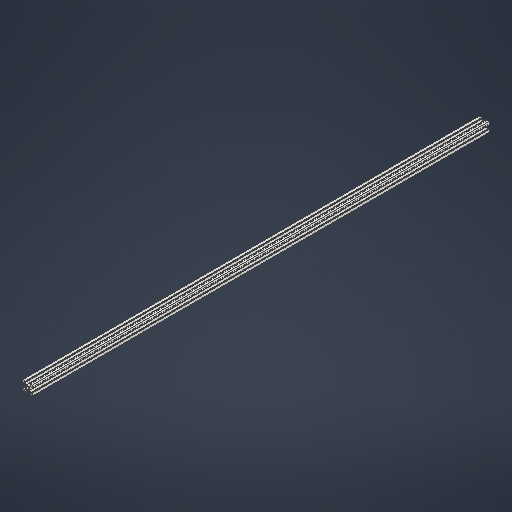
# Autodesk Inventor part: 铝方管2020x
Saved by Autodesk Inventor 2025 (Build 290162000, 162)
## iProperties
Created: 2025-06-18
Part Number: 铝方管2020x
Material: 常规
Document SubType Name: Modeling
Designer: XH
Density: 1 g/cm^3
Appearance: 默认
Author: XH
Autodesk Inventor part; units mm, degrees
ref_plane "YZ Plane" through (0, 0, 0) normal (1, 0, 0) x (0, 1, 0)
ref_plane "XZ Plane" through (0, 0, 0) normal (0, 1, 0) x (-1, 0, 0)
ref_plane "XY Plane" through (0, 0, 0) normal (0, 0, 1) x (1, 0, 0)
sketch "草图1" plane through (0, 0, 0) normal (0, 0, 1) x (1, 0, 0)
  line L0 (10, -10) -> (-10, -10)
  line L1 (-10, -10) -> (-10, 10)
  line L2 (-10, 10) -> (10, 10)
  line L3 (10, 10) -> (10, -10)
  line L4 (10, -10) -> (-10, 10) construction
  line L5 (-10, -10) -> (10, 10) construction
  point P0 (0, 0)
  dimension "d0" = 20
  dimension "d1" = 20
  constraints: 12 end point, 2 midpoint, 2 parallel, 1 horizontal, 1 perpendicular
  measures "d0" distance of L1.end L2.end
  measures "d1" distance of L0.end L1.end
extrude "拉伸1" add sketch "草图1" along normal blind 955
sketch "草图2" plane through (0, 0, 955) normal (0, 0, 1) x (1, 0, 0)
  circle A0 centre (0, 0) radius 2.55
  line L0 (-11.0615, 0) -> (0, 0)
  line L1 (0, 0) -> (0, 11.55)
  line L2 (-10, 10) -> (-10, -10)
  line L3 (10, 10) -> (-10, 10)
  line L4 (0, 3.9) -> (-3.9, 3.9)
  line L5 (-3.9, 3.9) -> (-3.9, 0)
  line L6 (-10, 10) -> (0, 0)
  line L7 (0, 1.0607) -> (-8.9393, 10)
  line L8 (-1.0607, 0) -> (-10, 8.9393)
  line L9 (-10, 10) -> (-3.1, 10)
  line L10 (-10, 3.1) -> (-10, 10)
  line L11 (-10, 10) -> (-3.65, 10)
  line L12 (-10, 3.65) -> (-10, 10)
  line L13 (-5.5, 12.0125) -> (-5.5, 5.5)
  line L14 (-10, 10) -> (-5.5, 10)
  line L15 (-5.5, 10) -> (-5.5, 5.5)
  line L16 (-5.5, 5.5) -> (-10, 5.5)
  line L17 (-10, 5.5) -> (-10, 10)
  line L18 (-5.5, 9.1) -> (0, 9.1)
  line L19 (-3.65, 10) -> (-3.65, 9.1)
  line L20 (-3.1, 10) -> (-3.1, 9.1)
  line L21 (-3.65, 9.6441) -> (-3.1, 9.6441)
  point P0 (-3.1, 9.55)
  point P1 (-2.8393, 3.9)
  point P2 (0, 10)
  point P3 (-5.5, 6.5607)
  dimension "d4" = 5.1
  dimension "d5" = 6.1
  dimension "d6" = 1.5
  dimension "d7" = 5.5
  dimension "d8" = 0.9
  dimension "d9" = 3.1
  dimension "d10" = 3.65
  constraints: 44 end point, 12 point on line, 7 perpendicular, 5 horizontal, 5 parallel, 2 coincident, 2 symmetric about line, 1 centre point, 1 midpoint, 1 vertical
  measures "d4" diameter of A0
  measures "d5" distance between parallel lines of L5 L2
  measures "d6" distance between parallel lines of L8 L7
  measures "d7" distance between parallel lines of L13 L1
  measures "d8" distance between parallel lines of L3 L18
  measures "d9" distance from line of point (-3.1, 9.55) L1
  measures "d10" distance between parallel lines of L19 L1
extrude "拉伸2" cut sketch "草图2" against normal up to surface (955 mm away) contours A0 L0 L1 | L1 L7 A0 | A0 L8 L0 | L7 L1 L6 A0 | L4 L7 L13 L18 L1 | A0 L6 L0 L8 | L18 L20 L3 L1 | L18 L19 L21 L20
mirror "镜像1" about plane through (0, 10, 955) normal (-1, 0, 0) of "拉伸2"
pattern_circular "环形阵列1" count 4 over 360 about axis through (0, 0, 955) along (0, 0, -1) of "拉伸2", "镜像1"
